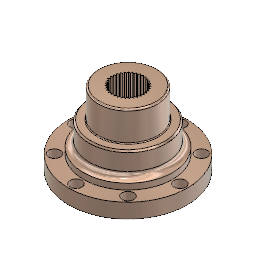
82a55af7-5d6a-4d23-acdf-7a3727aba519 (Autodesk Fusion 360 design; units mm, degrees)
Autodesk Fusion 360 part; units mm, degrees
sketch "Sketch1" plane through (0, 0, 0) normal (0, 0, 1) x (1, 0, 0)
  line L0 (40, 0) -> (40, 5)
  line L1 (40, 5) -> (35, 5)
  line L2 (35, 5) -> (35, 7)
  line L3 (35, 7) -> (33, 7)
  line L4 (33, 7) -> (33, 15)
  line L5 (33, 15) -> (30, 15)
  line L6 (30, 15) -> (30, 25)
  line L7 (30, 25) -> (25, 25)
  line L8 (20, 27) -> (20, -3)
  line L9 (25, 25) -> (25, 0)
  line L10 (25, 0) -> (40, 0)
  dimension "d3" = 5
  dimension "d6" = 5
  dimension "d7" = 2
  dimension "d8" = 2
  dimension "d9" = 8
  dimension "d10" = 10
  measures "d6" distance of origin
  measures "d10" distance of origin
revolve "Revolve1" add sketch "Sketch1" angle 360 about axis through (20, 27, 0) along (0, -1, 0)
fillet "Fillet1" radius 2 1 edges at (7.8797, 7, -4.701)
chamfer "Chamfer1" distance 0.5 angle 45 1 edges at (7.8797, 15, -4.701)
fillet "Fillet2" radius 0.5 1 edges at (10.6767, 25, -3.6162)
fillet "Fillet3" radius 0.25 1 edges at (10.6767, 15, -3.6162)
sketch "Sketch2" plane through (0, 5, 0) normal (0, 1, 0) x (-1, 0, 0)
  circle A0 centre (-20, 0) radius 15
  circle A1 centre (-20, 0) radius 20
  circle A2 centre (-2.5, 0) radius 2
  circle A3 centre (-7.6256, 12.3744) radius 2
  circle A4 centre (-20, 17.5) radius 2
  circle A5 centre (-32.3744, 12.3744) radius 2
  circle A6 centre (-37.5, 0) radius 2
  circle A7 centre (-32.3744, -12.3744) radius 2
  circle A8 centre (-20, -17.5) radius 2
  circle A9 centre (-7.6256, -12.3744) radius 2
  dimension "d16" = 4
  dimension "d18" = 360
  measures "d16" diameter of A2
extrude "Extrude1" cut sketch "Sketch2" against normal blind 7 contours A2 | A3 | A4 | A5 | A6 | A7 | A8 | A9
sketch "Sketch3" plane through (0, 25, 0) normal (0, 1, 0) x (-1, 0, 0)
  circle A0 centre (-20, 0) radius 5
  circle A1 centre (-20, 0) radius 9.5
  line L0 (-24.983, 0.4122) -> (-25.5, 0)
  line L1 (-25.5, 0) -> (-24.9828, -0.414)
  line L2 (-25.4116, -0.9821) -> (-24.8288, -1.297)
  line L3 (-24.9765, -0.4842) -> (-25.4116, -0.9821)
  line L4 (-25.1493, -1.9326) -> (-24.5196, -2.1384)
  line L5 (-24.8101, -1.365) -> (-25.1493, -1.9326)
  line L6 (-24.7215, -2.8209) -> (-24.0652, -2.9111)
  line L7 (-24.489, -2.2019) -> (-24.7215, -2.8209)
  line L8 (-24.1419, -3.6187) -> (-23.4801, -3.5902)
  line L9 (-24.0237, -2.9681) -> (-24.1419, -3.6187)
  line L10 (-23.4292, -4.3001) -> (-22.7831, -4.1538)
  line L11 (-23.4291, -3.6389) -> (-23.4292, -4.3001)
  line L12 (-22.6063, -4.8433) -> (-21.9967, -4.584)
  line L13 (-22.7243, -4.1927) -> (-22.6063, -4.8433)
  line L14 (-21.6996, -5.2308) -> (-21.1461, -4.8669)
  line L15 (-21.9318, -4.6117) -> (-21.6996, -5.2308)
  line L16 (-20.7383, -5.4502) -> (-20.2586, -4.9933)
  line L17 (-21.0773, -4.8826) -> (-20.7383, -5.4502)
  line L18 (-19.7532, -5.4945) -> (-19.3629, -4.9592)
  line L19 (-20.1882, -4.9965) -> (-19.7532, -5.4945)
  line L20 (-18.7761, -5.3621) -> (-18.4876, -4.7658)
  line L21 (-19.293, -4.9498) -> (-18.7761, -5.3621)
  line L22 (-17.8384, -5.0574) -> (-17.661, -4.4191)
  line L23 (-18.4206, -4.744) -> (-17.8384, -5.0574)
  line L24 (-16.9701, -4.5902) -> (-16.9095, -3.9305)
  line L25 (-17.5989, -4.3857) -> (-16.9701, -4.5902)
  line L26 (-16.1992, -3.9754) -> (-16.2573, -3.3155)
  line L27 (-16.8544, -3.8865) -> (-16.1992, -3.9754)
  line L28 (-15.5504, -3.2328) -> (-15.7255, -2.5939)
  line L29 (-16.211, -3.2624) -> (-15.5504, -3.2328)
  line L30 (-15.0447, -2.3864) -> (-15.331, -1.789)
  line L31 (-15.6893, -2.5334) -> (-15.0447, -2.3864)
  line L32 (-14.6982, -1.4632) -> (-15.0866, -0.9266)
  line L33 (-15.3063, -1.723) -> (-14.6982, -1.4632)
  line L34 (-14.5221, -0.493) -> (-15.0001, -0.0343)
  line L35 (-15.074, -0.8572) -> (-14.5221, -0.493)
  line L36 (-14.5221, 0.493) -> (-15.0743, 0.859)
  line L37 (-15.0001, 0.0361) -> (-14.5221, 0.493)
  line L38 (-14.6982, 1.4632) -> (-15.3069, 1.7247)
  line L39 (-15.0869, 0.9283) -> (-14.6982, 1.4632)
  line L40 (-15.0447, 2.3864) -> (-15.6902, 2.535)
  line L41 (-15.3316, 1.7907) -> (-15.0447, 2.3864)
  line L42 (-15.5504, 3.2328) -> (-16.2121, 3.2638)
  line L43 (-15.7264, 2.5954) -> (-15.5504, 3.2328)
  line L44 (-16.1992, 3.9754) -> (-16.8558, 3.8877)
  line L45 (-16.2585, 3.3168) -> (-16.1992, 3.9754)
  line L46 (-16.9701, 4.5902) -> (-17.6005, 4.3866)
  line L47 (-16.9109, 3.9316) -> (-16.9701, 4.5902)
  line L48 (-17.8384, 5.0574) -> (-18.4223, 4.7446)
  line L49 (-17.6625, 4.42) -> (-17.8384, 5.0574)
  line L50 (-18.7761, 5.3621) -> (-19.2948, 4.95)
  line L51 (-18.4893, 4.7663) -> (-18.7761, 5.3621)
  line L52 (-19.7532, 5.4945) -> (-20.19, 4.9964)
  line L53 (-19.3647, 4.9595) -> (-19.7532, 5.4945)
  line L54 (-20.7383, 5.4502) -> (-21.0791, 4.8822)
  line L55 (-20.2604, 4.9932) -> (-20.7383, 5.4502)
  line L56 (-21.6996, 5.2308) -> (-21.9335, 4.611)
  line L57 (-21.1478, 4.8665) -> (-21.6996, 5.2308)
  line L58 (-22.6063, 4.8433) -> (-22.7258, 4.1917)
  line L59 (-21.9983, 4.5833) -> (-22.6063, 4.8433)
  line L60 (-23.4292, 4.3001) -> (-23.4304, 3.6376)
  line L61 (-22.7846, 4.1529) -> (-23.4292, 4.3001)
  line L62 (-24.1419, 3.6187) -> (-24.0248, 2.9666)
  line L63 (-23.4813, 3.5889) -> (-24.1419, 3.6187)
  line L64 (-24.7215, 2.8209) -> (-24.4898, 2.2003)
  line L65 (-24.0662, 2.9096) -> (-24.7215, 2.8209)
  line L66 (-25.1493, 1.9326) -> (-24.8106, 1.3633)
  line L67 (-24.5204, 2.1368) -> (-25.1493, 1.9326)
  line L68 (-25.4116, 0.9821) -> (-24.9767, 0.4824)
  line L69 (-24.8293, 1.2953) -> (-25.4116, 0.9821)
  dimension "d22" = 360
extrude "Extrude2" cut sketch "Sketch3" against normal blind 35 contours A0 L36 L37 | A0 L34 L35 | A0 L38 L39 | A0 L32 L33 | A0 L40 L41 | A0 L30 L31 | A0 L42 L43 | A0 L28 L29 | A0 L44 L45 | A0 L26 L27 | A0 L46 L47 | A0 L24 L25 | A0 L48 L49 | A0 L22 L23 | A0 L50 L51 | A0 L20 L21 | A0 L52 L53 | A0 L18 L19 | A0 L54 L55 | A0 L16 L17 | A0 L56 L57 | A0 L14 L15 | A0 L58 L59 | A0 L12 L13 | A0 L60 L61 | A0 L10 L11 | A0 L62 L63 | A0 L8 L9 | A0 L64 L65 | A0 L6 L7 | A0 L66 L67 | A0 L4 L5 | A0 L68 L69 | A0 L2 L3 | A0 L0 L1
